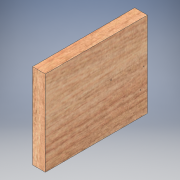
# Autodesk Inventor part: D1
Saved by Autodesk Inventor 2017 (Build 210142000, 142)
## iProperties
Created: 2017-02-12
Part Number: D1
Material: Generic
Document SubType Name: Modeling
Designer: kingb
Density: 1 g/cm^3
Appearance: Birch - Natural Polished
Author: kingb
Autodesk Inventor part; units mm, degrees
ref_plane "YZ Plane" through (0, 0, 0) normal (1, 0, 0) x (0, 1, 0)
ref_plane "XZ Plane" through (0, 0, 0) normal (0, 1, 0) x (-1, 0, 0)
ref_plane "XY Plane" through (0, 0, 0) normal (0, 0, 1) x (1, 0, 0)
sketch "Sketch1" plane through (0, 0, 0) normal (0, 0, 1) x (1, 0, 0)
  line L0 (0, 0) -> (19.05, 0)
  line L1 (19.05, 0) -> (19.05, 127)
  line L2 (19.05, 127) -> (0, 127)
  line L3 (0, 127) -> (0, 0)
  dimension "d0" = 19.05
  dimension "d1" = 127
  constraints: 8 end point, 2 parallel, 1 horizontal, 1 perpendicular
  measures "d0" distance of L2.end L1.end
  measures "d1" distance of L1.end L0.end
extrude "Extrusion1" add sketch "Sketch1" along normal blind 152.4
body "Solid1"
